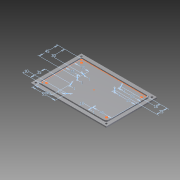
# Autodesk Inventor part: Base.Box.Lid
Saved by Autodesk Inventor 2011 (Build 150239000, 239)
## iProperties
Created: 2011-05-11
Part Number: Base.Box.Lid
Document SubType Name: Modeling
Designer: Rob
Density: 1 g/cm^3
Author: Rob
Autodesk Inventor part; units mm, degrees
ref_plane "YZ Plane" through (0, 0, 0) normal (1, 0, 0) x (0, 1, 0)
ref_plane "XZ Plane" through (0, 0, 0) normal (0, 1, 0) x (-1, 0, 0)
ref_plane "XY Plane" through (0, 0, 0) normal (0, 0, 1) x (1, 0, 0)
sketch "Sketch1" plane through (0, 0, 0) normal (0, 0, 1) x (1, 0, 0)
  line L0 (-83, 53) -> (83, 53) construction
  line L1 (83, 53) -> (83, -53) construction
  line L2 (83, -53) -> (-83, -53) construction
  line L3 (-83, -53) -> (-83, 53) construction
  line L4 (-83, 53) -> (83, -53) construction
  line L5 (83, 53) -> (-83, -53) construction
  line L6 (-91, 61) -> (91, 61)
  line L7 (91, 61) -> (91, -61)
  line L8 (91, -61) -> (-91, -61)
  line L9 (-91, -61) -> (-91, 61)
  line L10 (-91, 61) -> (91, -61) construction
  line L11 (-91, -61) -> (91, 61) construction
  point P0 (0, 0)
  point P1 (0, 0)
  point P2 (0, 0)
  dimension "d0" = 166
  dimension "d1" = 106
  dimension "d2" = 8
  dimension "d3" = 8
  constraints: 24 end point, 4 parallel, 3 midpoint, 2 horizontal, 2 perpendicular, 1 coincident
  measures "d0" distance of L1.end L2.end
  measures "d1" distance of L0.end L1.end
  measures "d2" distance between parallel lines of L3 L9
  measures "d3" distance between parallel lines of L0 L6
extrude "Extrusion1" add sketch "Sketch1" along normal blind 3
sketch "Sketch2" plane through (0, 0, 3) normal (0, 0, 1) x (1, 0, 0)
  line L0 (-83, 53) -> (83, 53)
  line L1 (83, 53) -> (83, -53)
  line L2 (83, -53) -> (-83, -53)
  line L3 (-83, -53) -> (-83, 53)
  line L4 (-83, 53) -> (83, -53) construction
  line L5 (83, 53) -> (-83, -53) construction
  line L6 (-80, 50) -> (80, 50)
  line L7 (80, 50) -> (80, -50)
  line L8 (80, -50) -> (-80, -50)
  line L9 (-80, -50) -> (-80, 50)
  line L10 (-80, -50) -> (80, 50) construction
  line L11 (80, -50) -> (-80, 50) construction
  point P0 (0, 0)
  point P1 (0, 0)
  point P2 (0, 0)
  dimension "d6" = 166
  dimension "d7" = 106
  dimension "d8" = 3
  dimension "d9" = 3
  constraints: 24 end point, 4 parallel, 3 midpoint, 2 horizontal, 2 perpendicular, 1 coincident
  measures "d6" distance of L1.end L2.end
  measures "d7" distance of L0.end L1.end
  measures "d8" distance between parallel lines of L0 L6
  measures "d9" distance between parallel lines of L1 L7
extrude "Extrusion2" add sketch "Sketch2" along normal blind 3
fillet "Fillet1" radius 3 4 edges at (80, 50, 4.5) (80, -50, 4.5) (-80, -50, 4.5) (-80, 50, 4.5)
fillet "Fillet2" radius 6 4 edges at (83, 53, 4.5) (83, -53, 4.5) (-83, -53, 4.5) (-83, 53, 4.5)
sketch "Sketch3" plane through (0, 0, 0) normal (0, 0, -1) x (-1, 0, 0)
  line L0 (91, 61) -> (-91, 61) projected
  line L1 (-91, 61) -> (-91, -61) projected
  line L2 (91, -61) -> (91, 61) projected
  circle A0 centre (-85, 55) radius 2
  line L3 (0, 0) -> (-15.5328, 0) construction
  line L4 (0, 0) -> (0, 8.2904) construction
  circle A1 centre (-85, -55) radius 2
  circle A2 centre (85, 55) radius 2
  circle A3 centre (85, -55) radius 2
  dimension "d14" = 4
  dimension "d15" = 6
  dimension "d16" = 6
  constraints: 4 centre point, 4 end point, 3 symmetric about line, 2 perpendicular, 3 other
  measures "d14" diameter of A0
  measures "d15" distance from line of L0 A0.centre
  measures "d16" distance from line of L1 A0.centre
hole "Hole1" at (85, 55, 0) at (85, -55, 0) at (-85, -55, 0) at (-85, 55, 0) direction (0, 0, 1) diameter 4.5 depth 8 tip angle 118 clearance for "Flat Head Machine Screw" size "M4" standard "Ansi Metric M Profile"
sketch "Sketch4" plane through (0, 0, 3) normal (0, 0, 1) x (1, 0, 0)
  line L0 (-80, 47) -> (-80, -47) projected
  line L1 (-77, -50) -> (77, -50) projected
  line L2 (77, 50) -> (-77, 50) projected
  line L3 (0, 0) -> (-11.513, 0) construction
  line L4 (0, 0) -> (0, -7.6384) construction
  circle A0 centre (-72, -42) radius 5.1497
  circle A1 centre (-72, 42) radius 5.1497
  circle A2 centre (72, -42) radius 5.1497
  circle A3 centre (72, 42) radius 5.1497
  dimension "d24" = 8
  dimension "d25" = 8
  constraints: 4 centre point, 4 end point, 3 symmetric about line, 1 parallel, 1 perpendicular, 3 other
  measures "d24" distance from line of L0 A0.centre
  measures "d25" distance from line of L1 A0.centre
hole "Hole2" at (-72, -42, 3) at (-72, 42, 3) at (72, -42, 3) at (72, 42, 3) direction (0, 0, -1) diameter 4.5 depth 8 tip angle 118 clearance for "Flat Head Machine Screw" size "M4" standard "Ansi Metric M Profile"
sketch "Sketch5" plane through (0, 0, 3) normal (0, 0, 1) x (1, 0, 0)
  circle A0 centre (72, 42) radius 2.25 projected
  circle A1 centre (72, -42) radius 2.25 projected
  circle A2 centre (-72, 42) radius 2.25 projected
  circle A3 centre (-72, -42) radius 2.25 projected
  arc A4 (-77, 50) -> (-80, 47) centre (-77, 47) ccw projected
  line L0 (-80, 47) -> (-80, -47) projected
  arc A5 (-80, -47) -> (-77, -50) centre (-77, -47) ccw projected
  line L1 (-77, -50) -> (77, -50) projected
  arc A6 (77, -50) -> (80, -47) centre (77, -47) ccw projected
  line L2 (80, -47) -> (80, 47) projected
  arc A7 (80, 47) -> (77, 50) centre (77, 47) ccw projected
  line L3 (77, 50) -> (-77, 50) projected
  circle A8 centre (-25, -40) radius 0.5
  circle A9 centre (-40, -15) radius 0.5
  circle A10 centre (-45, 5) radius 0.5
  circle A11 centre (-45, 20) radius 0.5
  circle A12 centre (35, -40) radius 0.5
  circle A13 centre (25, 25) radius 0.5
  circle A14 centre (25, 40) radius 0.5
  point P0 (0, 0)
  dimension "d33" = 1
  dimension "d34" = 1
  dimension "d35" = 1
  dimension "d36" = 1
  dimension "d37" = 1
  dimension "d38" = 1
  dimension "d39" = 1
  dimension "d41" = 55
  dimension "d43" = 40
  dimension "d44" = 35
  dimension "d45" = 35
  dimension "d50" = 55
  dimension "d51" = 55
  dimension "d53" = 45
  dimension "d54" = 30
  dimension "d55" = 45
  dimension "d56" = 35
  dimension "d57" = 10
  dimension "d58" = 10
  dimension "d59" = 25
  dimension "d60" = 10
  constraints: 7 centre point
  measures "d33" diameter of A8
  measures "d34" diameter of A9
  measures "d35" diameter of A10
  measures "d36" diameter of A11
  measures "d37" diameter of A12
  measures "d38" diameter of A13
  measures "d39" diameter of A14
  measures "d41" distance from line of L0 A8.centre
  measures "d43" distance from line of L0 A9.centre
  measures "d44" distance from line of L0 A10.centre
  measures "d45" distance from line of L0 A11.centre
  measures "d50" distance from line of L2 A14.centre
  measures "d51" distance from line of L2 A13.centre
  measures "d53" distance from line of L2 A12.centre
  measures "d54" distance from line of L3 A11.centre
  measures "d55" distance from line of L3 A10.centre
  measures "d56" distance from line of L1 A9.centre
  measures "d57" distance from line of L1 A8.centre
  measures "d58" distance from line of L3 A14.centre
  measures "d59" distance from line of L3 A13.centre
  measures "d60" distance from line of L1 A12.centre
equation "\"d15\" = 1.5 * d14"
equation "\"d16\" = 1.5 * d14"
body "Solid1"
